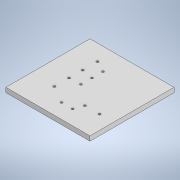
# Autodesk Inventor part: sheetmetalbottom
Saved by Autodesk Inventor 2020.2 (Build 242310000, 310)
## iProperties
Created: 2020-02-05
Part Number: sheetmetalbottom
Material: Generic
Document SubType Name: Modeling
Designer: ColinP
Density: 1 g/cm^3
Appearance: Default
Author: ColinP
Autodesk Inventor part; units mm, degrees
ref_plane "YZ Plane" through (0, 0, 0) normal (1, 0, 0) x (0, 1, 0)
ref_plane "XZ Plane" through (0, 0, 0) normal (0, 1, 0) x (-1, 0, 0)
ref_plane "XY Plane" through (0, 0, 0) normal (0, 0, 1) x (1, 0, 0)
sketch "Sketch1" plane through (0, 0, 0) normal (0, 1, 0) x (-1, 0, 0)
  line L0 (114.3, 114.3) -> (-114.3, 114.3)
  line L1 (-114.3, 114.3) -> (-114.3, -114.3)
  line L2 (-114.3, -114.3) -> (114.3, -114.3)
  line L3 (114.3, -114.3) -> (114.3, 114.3)
  point P0 (0, 0)
  dimension "d0" = 228.6
  dimension "d1" = 228.6
  constraints: 8 end point, 2 parallel, 1 horizontal, 1 perpendicular
  measures "d0" distance of L2.end L1.end
  measures "d1" distance of L1.end L0.end
extrude "Extrusion1" add sketch "Sketch1" along normal blind 12.7
sketch "Sketch2" plane through (0, 12.7, 0) normal (0, -1, 0) x (1, 0, 0)
  line L0 (114.3, -114.3) -> (-114.3, -114.3) projected
  line L1 (-114.3, -114.3) -> (-50.292, -114.3)
  line L2 (-50.292, -114.3) -> (-50.292, -70.358)
  line L3 (-50.292, -70.358) -> (-50.292, -30.353)
  line L4 (-50.292, -30.353) -> (-50.292, 6.731)
  line L5 (-50.292, 6.731) -> (-50.292, 46.736)
  point P0 (0, 0)
  dimension "d4" = 64.008
  dimension "d5" = 43.942
  dimension "d6" = 40.005
  dimension "d7" = 37.084
  dimension "d8" = 40.005
  constraints: 10 end point, 4 point on line, 1 perpendicular
  measures "d4" distance of L0.end L1.end
  measures "d5" distance of L1.end L2.end
  measures "d6" distance of L2.end L3.end
  measures "d7" distance of L3.end L4.end
  measures "d8" distance of L4.end L5.end
hole "Hole1" at (-50.292, 12.7, 46.736) at (-50.292, 12.7, 6.731) at (-50.292, 12.7, -30.353) at (-50.292, 12.7, -70.358) direction (0, -1, 0) diameter 3.556 depth 25.4 counterbore diameter 6.096 counterbore depth 4.064
sketch "Sketch3" plane through (0, 0, 0) normal (0, -1, 0) x (1, 0, 0)
  line L0 (-114.3, -114.3) -> (-19.304, -114.3)
  line L1 (114.3, -114.3) -> (-114.3, -114.3) projected
  line L2 (-19.304, -114.3) -> (-19.304, -54.356)
  line L3 (-19.304, -54.356) -> (-19.304, -24.384)
  line L4 (-19.304, -24.384) -> (-19.304, 5.588)
  line L5 (114.3, 114.3) -> (63.5, 114.3)
  line L6 (-114.3, 114.3) -> (114.3, 114.3) projected
  line L7 (63.5, 114.3) -> (63.5, 74.422)
  line L8 (63.5, 74.422) -> (33.528, 74.422)
  line L9 (63.5, 114.3) -> (63.5, 74.422)
  line L10 (63.5, 74.422) -> (33.528, 74.422)
  line L11 (33.528, 74.422) -> (27.178, 74.422)
  line L12 (27.178, 74.422) -> (-2.794, 74.422)
  point P0 (0, 0)
  dimension "d16" = 94.996
  dimension "d17" = 59.944
  dimension "d18" = 29.972
  dimension "d19" = 29.972
  dimension "d20" = 50.8
  dimension "d21" = 39.878
  dimension "d22" = 29.972
  dimension "d23" = 39.878
  dimension "d24" = 6.35
  dimension "d25" = 29.972
  constraints: 22 end point, 6 point on line, 4 perpendicular, 1 vertical
  measures "d16" distance of L0.start L0.end
  measures "d17" distance of L0.end L2.end
  measures "d18" distance of L2.end L3.end
  measures "d19" distance of L3.end L4.end
  measures "d20" distance of L5.start L5.end
  measures "d21" distance of L5.end L7.end
  measures "d22" distance of L7.end L8.end
  measures "d23" distance of L5.end L9.end
  measures "d24" distance of L10.end L11.end
  measures "d25" distance of L11.end L12.end
hole "Hole2" at (-2.794, 0, 74.422) at (27.178, 0, 74.422) at (-19.304, 0, 5.588) at (-19.304, 0, -24.384) at (-19.304, 0, -54.356) direction (0, 1, 0) diameter 5.842 depth 25.4
sketch "Sketch4" plane through (0, 12.7, 0) normal (0, 1, 0) x (1, 0, 0)
  line L0 (114.3, -114.3) -> (76.2, -114.3)
  line L1 (-114.3, -114.3) -> (114.3, -114.3) projected
  line L2 (76.2, -114.3) -> (76.2, -50.292)
  line L3 (76.2, -50.292) -> (36.322, -50.292)
  point P0 (0, 0)
  dimension "d33" = 38.1
  dimension "d34" = 64.008
  dimension "d35" = 39.878
  constraints: 6 end point, 1 horizontal, 1 perpendicular, 1 point on line
  measures "d33" distance of L0.start L0.end
  measures "d34" distance of L0.end L2.end
  measures "d35" distance of L2.end L3.end
hole "Hole3" at (76.2, 12.7, 50.292) at (36.322, 12.7, 50.292) direction (0, -1, 0) diameter 3.556 depth 25.4 counterbore diameter 6.096 counterbore depth 4.064
sketch "Sketch5" plane through (0, 12.7, 0) normal (0, 1, 0) x (1, 0, 0)
  line L0 (114.3, 114.3) -> (-114.3, 114.3) projected
  line L1 (-114.3, 114.3) -> (-104.14, 114.3)
  line L2 (-104.14, 114.3) -> (-114.3, 114.3)
  line L3 (-104.14, 114.3) -> (-104.14, 50.8)
  line L4 (-104.14, 50.8) -> (-104.14, -12.7)
  line L5 (-104.14, -12.7) -> (-104.14, -76.2)
  line L6 (-114.3, 114.3) -> (-114.3, 104.14)
  line L7 (-114.3, 114.3) -> (-114.3, -114.3) projected
  line L8 (-114.3, 104.14) -> (-50.8, 104.14)
  line L9 (-50.8, 104.14) -> (12.7, 104.14)
  line L10 (12.7, 104.14) -> (76.2, 104.14)
  line L11 (-114.3, -114.3) -> (114.3, -114.3) projected
  line L12 (114.3, -114.3) -> (114.3, -104.14)
  line L13 (114.3, -114.3) -> (114.3, 114.3) projected
  line L14 (114.3, -104.14) -> (50.8, -104.14)
  line L15 (50.8, -104.14) -> (-12.7, -104.14)
  line L16 (-12.7, -104.14) -> (-76.2, -104.14)
  line L17 (114.3, -114.3) -> (104.14, -114.3)
  line L18 (104.14, -114.3) -> (104.14, -50.8)
  line L19 (104.14, -50.8) -> (104.14, 12.7)
  line L20 (104.14, 12.7) -> (104.14, 76.2)
  point P0 (0, 0)
  dimension "d43" = 10.16
  dimension "d44" = 63.5
  dimension "d45" = 63.5
  dimension "d46" = 63.5
  dimension "d47" = 10.16
  dimension "d48" = 63.5
  dimension "d49" = 90
  dimension "d50" = 63.5
  dimension "d51" = 63.5
  dimension "d52" = 10.16
  dimension "d53" = 63.5
  dimension "d54" = 63.5
  dimension "d55" = 63.5
  dimension "d56" = 10.16
  dimension "d57" = 63.5
  dimension "d58" = 63.5
  dimension "d59" = 63.5
  constraints: 34 end point, 12 point on line, 3 perpendicular, 1 collinear, 1 vertical
  measures "d43" distance of L0.end L1.end
  measures "d44" distance of L1.end L3.end
  measures "d45" distance of L3.end L4.end
  measures "d46" distance of L4.end L5.end
  measures "d47" distance of L0.end L6.end
  measures "d48" distance of L6.end L8.end
  measures "d49" angle of L8 L6
  measures "d50" distance of L8.end L9.end
  measures "d51" distance of L9.end L10.end
  measures "d52" distance of L11.end L12.end
  measures "d53" distance of L12.end L14.end
  measures "d54" distance of L14.end L15.end
  measures "d55" distance of L15.end L16.end
  measures "d56" distance of L11.end L17.end
  measures "d57" distance of L17.end L18.end
  measures "d58" distance of L18.end L19.end
  measures "d59" distance of L19.end L20.end
hole "Hole4" [suppressed]
body "Solid1"
